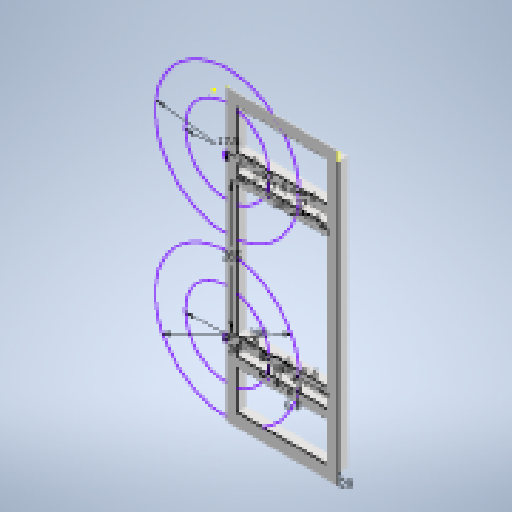
# Autodesk Inventor part: DOF10
Saved by Autodesk Inventor 2024 (Build 280153000, 153)
## iProperties
Created: 2024-10-16
Part Number: DOF10
Material: 一般
Document SubType Name: Modeling
Designer: jerry
Density: 1 g/cm^3
Appearance: 預設
Author: jerry
Autodesk Inventor part; units mm, degrees
ref_plane "YZ Plane" through (0, 0, 0) normal (1, 0, 0) x (0, 1, 0)
ref_plane "XZ Plane" through (0, 0, 0) normal (0, 1, 0) x (-1, 0, 0)
ref_plane "XY Plane" through (0, 0, 0) normal (0, 0, 1) x (1, 0, 0)
sketch "草圖1" plane through (0, 0, 0) normal (0, 0, 1) x (1, 0, 0)
  line L0 (0, 0) -> (25, 0)
  line L1 (25.6094, 0) -> (25.6094, 20)
  line L2 (25.6094, 20) -> (250.6094, 20)
  line L3 (250.6094, 20) -> (250.6094, -565)
  line L4 (250.6094, -565) -> (25.6094, -565)
  line L5 (25.6094, -565) -> (25.6094, 20)
  line L6 (25.6094, 0) -> (25.6094, -5)
  line L7 (45.6094, -5) -> (230.6094, -5)
  line L8 (230.6094, -5) -> (230.6094, -85)
  line L9 (230.6094, -85) -> (45.6094, -85)
  line L10 (45.6094, -85) -> (45.6094, -5)
  line L11 (45.6094, -102.5) -> (230.6094, -102.5)
  line L12 (230.6094, -102.5) -> (230.6094, -122.5)
  line L13 (230.6094, -122.5) -> (45.6094, -122.5)
  line L14 (45.6094, -122.5) -> (45.6094, -102.5)
  line L15 (45.6094, -140) -> (230.6094, -140)
  line L16 (230.6094, -140) -> (230.6094, -405)
  line L17 (230.6094, -405) -> (45.6094, -405)
  line L18 (45.6094, -405) -> (45.6094, -140)
  line L19 (45.6094, -422.5) -> (230.6094, -422.5)
  line L20 (230.6094, -422.5) -> (230.6094, -442.5)
  line L21 (230.6094, -442.5) -> (45.6094, -442.5)
  line L22 (45.6094, -442.5) -> (45.6094, -422.5)
  line L23 (45.6094, -460) -> (230.6094, -460)
  line L24 (230.6094, -460) -> (230.6094, -540)
  line L25 (230.6094, -540) -> (45.6094, -540)
  line L26 (45.6094, -540) -> (45.6094, -460)
  dimension "d0" = 25
  dimension "d1" = 20
  dimension "d2" = 225
  dimension "d3" = 585
  dimension "d4" = 5
  dimension "d6" = 20
  dimension "d9" = 185
  dimension "d10" = 80
  dimension "d11" = 185
  dimension "d13" = 185
  dimension "d14" = 20
  dimension "d16" = 185
  dimension "d17" = 265
  dimension "d19" = 185
  dimension "d20" = 20
  dimension "d22" = 185
  dimension "d23" = 80
  constraints: 54 end point, 10 parallel, 8 perpendicular, 6 horizontal, 2 point on line, 1 vertical
  measures "d0" distance of L0.start L0.end
  measures "d1" distance of L1.start L1.end
  measures "d2" distance of L3.end L4.end
  measures "d3" distance of L2.end L3.end
  measures "d4" distance of L1.start L6.end
  measures "d6" distance of L6.end L7.start
  measures "d9" distance of L7.start L7.end
  measures "d10" distance of L7.end L8.end
  measures "d11" distance of L8.end L9.end
  measures "d13" distance of L12.end L13.end
  measures "d14" distance of L11.end L12.end
  measures "d16" distance of L16.end L17.end
  measures "d17" distance of L15.end L16.end
  measures "d19" distance of L20.end L21.end
  measures "d20" distance of L19.end L20.end
  measures "d22" distance of L24.end L25.end
  measures "d23" distance of L23.end L24.end
extrude "擠出1" add sketch "草圖1" along normal blind 2
sketch "草圖2" plane through (0, 0, 0) normal (0, 0, -1) x (-1, 0, 0)
  line L0 (-250.6094, -565) -> (-250.6094, 20) projected
  line L1 (-250.6094, -565) -> (-250.6094, -545)
  line L2 (-25.6094, 20) -> (-25.6094, -565) projected
  line L3 (-250.6094, -545) -> (-25.6094, -545)
  line L4 (-25.6094, -545) -> (-25.6094, 0)
  line L5 (-25.6094, 0) -> (-250.6094, 0)
  line L6 (-250.6094, 0) -> (-250.6094, -545)
  line L7 (-230.6094, -460) -> (-230.6094, -540) projected
  line L8 (-45.6094, -540) -> (-45.6094, -460) projected
  line L9 (-230.6094, -540) -> (-45.6094, -540)
  line L10 (-45.6094, -540) -> (-45.6094, -460)
  line L11 (-45.6094, -460) -> (-230.6094, -460)
  line L12 (-230.6094, -460) -> (-230.6094, -540)
  line L13 (-230.6094, -442.5) -> (-45.6094, -442.5) projected
  line L14 (-230.6094, -442.5) -> (-45.6094, -442.5)
  line L15 (-45.6094, -442.5) -> (-45.6094, -422.5)
  line L16 (-45.6094, -422.5) -> (-230.6094, -422.5)
  line L17 (-230.6094, -422.5) -> (-230.6094, -442.5)
  line L18 (-230.6094, -405) -> (-45.6094, -405) projected
  line L19 (-230.6094, -405) -> (-45.6094, -405)
  line L20 (-45.6094, -405) -> (-45.6094, -140)
  line L21 (-45.6094, -140) -> (-230.6094, -140)
  line L22 (-230.6094, -140) -> (-230.6094, -405)
  line L23 (-230.6094, -122.5) -> (-45.6094, -122.5) projected
  line L24 (-45.6094, -102.5) -> (-230.6094, -102.5) projected
  line L25 (-230.6094, -122.5) -> (-45.6094, -122.5)
  line L26 (-45.6094, -122.5) -> (-45.6094, -102.5)
  line L27 (-45.6094, -102.5) -> (-230.6094, -102.5)
  line L28 (-230.6094, -102.5) -> (-230.6094, -122.5)
  line L29 (-230.6094, -85) -> (-45.6094, -85) projected
  line L30 (-45.6094, -5) -> (-230.6094, -5) projected
  line L31 (-230.6094, -85) -> (-45.6094, -85)
  line L32 (-45.6094, -85) -> (-45.6094, -5)
  line L33 (-45.6094, -5) -> (-230.6094, -5)
  line L34 (-230.6094, -5) -> (-230.6094, -85)
  circle A0 centre (-25.6094, -102.5) radius 8.75
  line L35 (-25.6094, 20) -> (-25.6094, -565) projected
  circle A1 centre (-25.6094, -93.75) radius 85
  circle A2 centre (-25.6094, -93.75) radius 145
  circle A3 centre (-170.6094, -93.75) radius 3
  circle A4 centre (-110.6094, -93.75) radius 3
  line L36 (-170.6094, -93.75) -> (-170.6094, -130.75)
  line L37 (-110.6094, -93.75) -> (-110.6094, -130.75)
  circle A5 centre (-110.6094, -130.75) radius 3
  circle A6 centre (-170.6094, -130.75) radius 3
  circle A7 centre (-25.6094, -422.5) radius 8.75
  circle A8 centre (-25.6094, -413.75) radius 85
  circle A9 centre (-25.6094, -413.75) radius 145
  circle A10 centre (-170.6094, -413.75) radius 3
  circle A11 centre (-110.6094, -413.75) radius 3
  line L38 (-110.6094, -413.75) -> (-110.6094, -450.75)
  line L39 (-170.6094, -413.75) -> (-170.6094, -450.75)
  circle A12 centre (-170.6094, -450.75) radius 3
  circle A13 centre (-110.6094, -450.75) radius 3
  point P0 (0, 0)
  dimension "d33" = 17.5
  dimension "d34" = 170
  dimension "d35" = 290
  dimension "d42" = 17.5
  dimension "d43" = 170
  dimension "d44" = 290
  dimension "d26" = 20
  dimension "d27" = 185
  dimension "d28" = 20
  dimension "d29" = 185
  dimension "d30" = 265
  dimension "d36" = 6
  dimension "d37" = 6
  dimension "d38" = 37
  dimension "d39" = 37
  dimension "d40" = 6
  dimension "d41" = 6
  dimension "d45" = 6
  dimension "d46" = 6
  dimension "d47" = 37
  dimension "d48" = 6
  dimension "d49" = 6
  constraints: 58 end point, 12 parallel, 8 centre point, 7 perpendicular, 6 coincident, 6 horizontal, 6 point on line, 5 vertical, 4 horizontal alignment, 2 vertical alignment, 12 other
  measures "d26" distance of L0.start L1.end
  measures "d27" distance of L16.end L15.end
  measures "d28" distance of L15.end L14.end
  measures "d29" distance of L21.end L20.end
  measures "d30" distance of L20.end L19.end
  measures "d36" diameter of A3
  measures "d37" diameter of A4
  measures "d38" distance of L36.start L36.end
  measures "d39" distance of L37.start L37.end
  measures "d40" diameter of A5
  measures "d41" diameter of A6
  measures "d45" diameter of A10
  measures "d46" diameter of A11
  measures "d47" distance of L38.start L38.end
  measures "d48" diameter of A12
  measures "d49" diameter of A13
extrude "擠出2" add sketch "草圖2" along normal blind 20 contours A12 | A6 | L0 L5 A2 L30 L34 L29 A3 L36 L24 L28 L23 L21 L22 L18 A9 A10 L39 L16 L17 L13 L11 L7 L9 L3 | A9 L9 L8 A8 L2 L3 | L5 L2 A1 L32 L30 A2 | A8 L8 L11 L13 L15 L16 A11 L18 L20 L2 A7 | A13 | A9 L13 A8 L11 | L2 A0 A1 L20 L21 L23 L26 L24 A4 L29 L32 | A2 L20 A1 L2 | L2 A9 L20 A2 | L29 A1 A4 L37 L24 A2 A3 | A7 L2 | L2 A8 L20 A9 | L2 A0 | A3 A2 | A2 L36 A3 | A9 A10 L18 A8 A11 L38 L16 | L16 L39 A10 A9 | A5 | A2 L23 A1 L21 | A4 A1 | A1 L37 A4 | A2 A3 L36 | A3 A2 L24 L36 | L16 L38 A11 A8 | A10 L39 A9 | A9 A10 | A1 A4 L37 | A4 A1 L24 L37 | A11 L38 A8 | A8 A11 | A10 A9 L39 | A11 A8 L38 picked at (-27.5435, -424.6832) picked at (-30.39, -103.7836)
extrude "擠出3" cut sketch "草圖2" along normal through all both and the other way through all contours A12 | A6 | A13 | A3 A2 | A2 L36 A3 | A5 | A4 A1 | A1 L37 A4 | A2 A3 L36 | A10 L39 A9 | A9 A10 | A1 A4 L37 | A11 L38 A8 | A8 A11 | A10 A9 L39 | A11 A8 L38
